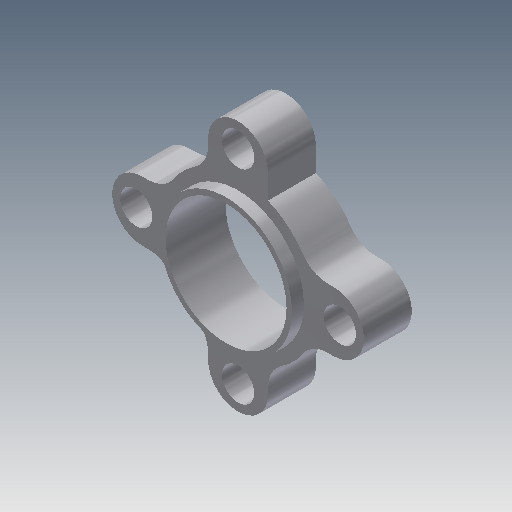
# Autodesk Inventor part: リンク_ふくらはぎ_サブフレーム_1_4
Saved by Autodesk Inventor 2017.3 (Build 213256000, 256)
## iProperties
Created: 2016-05-04
Part Number: リンク_ふくらはぎ_サブフレーム_1_4
Material: アルミニウム 2014-T4
Document SubType Name: Modeling
Designer: hiroaki
Density: 2.8 g/cm^3
Appearance: サテン
Mass: 1.21286 g
Surface Area: 8.00799 cm^2
Volume: 0.433165 cm^3
Author: hiroaki
Autodesk Inventor part; units mm, degrees
ref_plane "YZ Plane" through (0, 0, 0) normal (1, 0, 0) x (0, 1, 0)
ref_plane "XZ Plane" through (0, 0, 0) normal (0, 1, 0) x (-1, 0, 0)
ref_plane "XY Plane" through (0, 0, 0) normal (0, 0, 1) x (1, 0, 0)
sketch "スケッチ1" plane through (0, 0, 0) normal (0, 0, 1) x (1, 0, 0)
  circle A0 centre (0, 0) radius 10.5
  circle A1 centre (0, 0) radius 5.05
  circle A2 centre (0, 8.5) radius 1.35
  circle A3 centre (-6.0104, 6.0104) radius 1.04
  line L0 (0, 8.5) -> (0, 0) construction
  line L1 (0, 0) -> (-6.0104, 6.0104) construction
  circle A4 centre (0, 0) radius 8.5 construction
  circle A5 centre (-8.5, 0) radius 1.35
  circle A6 centre (-6.0104, -6.0104) radius 1.04
  circle A7 centre (0, -8.5) radius 1.35
  circle A8 centre (6.0104, -6.0104) radius 1.04
  circle A9 centre (8.5, 0) radius 1.35
  circle A10 centre (6.0104, 6.0104) radius 1.04
  dimension "d0" = 21
  dimension "d1" = 10.1
  dimension "d2" = 2.7
  dimension "d3" = 45
  dimension "d4" = 2.08
  dimension "d5" = 17
  dimension "d8" = 360
  constraints: 11 centre point, 4 coincident, 4 end point, 2 point on circle, 1 vertical, 1 vertical alignment, 17 other
  measures "d0" diameter of A0
  measures "d1" diameter of A1
  measures "d2" diameter of A2
  measures "d3" angle of L1 L0
  measures "d4" diameter of A3
  measures "d5" diameter of A4
extrude "押し出し1" add sketch "スケッチ1" along normal blind 4 contours A0 | A3 | A6 | A8 | A10
sketch "スケッチ2" plane through (0, 0, 4) normal (0, 0, 1) x (1, 0, 0)
  circle A0 centre (0, 0) radius 5.05 projected
  circle A1 centre (0, 0) radius 10.5 projected
  circle A2 centre (0, 0) radius 5.5
  dimension "d12" = 11
  constraints: 1 centre point, 1 coincident
  measures "d12" diameter of A2
extrude "押し出し2" add sketch "スケッチ2" along normal blind 1 contours A2
sketch "スケッチ4" plane through (0, 0, 4) normal (0, 0, 1) x (1, 0, 0)
  circle A0 centre (0, 0) radius 5.5 projected
  circle A1 centre (-8.5, 0) radius 1.35 projected
  circle A2 centre (0, 8.5) radius 1.35 projected
  circle A3 centre (0, 0) radius 10.5 projected
  line L0 (0, 8.5) -> (0, 0) construction
  line L1 (0, 0) -> (-8.5, 0) construction
  line L2 (0, 0) -> (-7.4246, 7.4246) construction
  circle A4 centre (0, 0) radius 10.5 construction
  line L3 (-12.2474, 2.5) -> (-6, 2.5)
  line L4 (-2.5, 6) -> (-2.5, 12.2474)
  arc A5 (-2.5, 12.2474) -> (-12.2474, 2.5) centre (0, 0) ccw
  arc A6 (-2.5, 6) -> (-6, 2.5) centre (0, 0) ccw
  circle A7 centre (0, 0) radius 5.5 projected
  line L5 (-2.5, -12.2474) -> (-2.5, -6)
  line L6 (-6, -2.5) -> (-12.2474, -2.5)
  arc A8 (-12.2474, -2.5) -> (-2.5, -12.2474) centre (0, 0) ccw
  arc A9 (-6, -2.5) -> (-2.5, -6) centre (0, 0) ccw
  line L7 (12.2474, -2.5) -> (6, -2.5)
  line L8 (2.5, -6) -> (2.5, -12.2474)
  arc A10 (2.5, -12.2474) -> (12.2474, -2.5) centre (0, 0) ccw
  arc A11 (2.5, -6) -> (6, -2.5) centre (0, 0) ccw
  line L9 (2.5, 12.2474) -> (2.5, 6)
  line L10 (6, 2.5) -> (12.2474, 2.5)
  arc A12 (12.2474, 2.5) -> (2.5, 12.2474) centre (0, 0) ccw
  arc A13 (6, 2.5) -> (2.5, 6) centre (0, 0) ccw
  dimension "d24" = 45
  dimension "d25" = 2.5
  dimension "d26" = 2.5
  dimension "d27" = 2
  dimension "d30" = 360
  dimension "d35" = 1
  constraints: 22 end point, 16 point on circle, 8 centre point, 2 coincident, 2 vertical, 1 horizontal, 1 perpendicular, 45 other
  measures "d24" angle of L0 L2
  measures "d25" distance between parallel lines of L1 L3
  measures "d26" distance between parallel lines of L0 L4
  measures "d35" radial gap between concentric circles of A0 A6
extrude "押し出し4" cut sketch "スケッチ4" against normal blind 10 contours L10 A13 L9 A3 | A3 L9 A12 L10 | L7 A10 L8 A3 | A3 L8 A11 L7 | L4 A6 L3 A3 | A3 L3 A5 L4 | L5 A8 L6 A3 | A3 L6 A9 L5
fillet "フィレット2" radius 2.5 15 edges at (2.5, -6, 2) (2.5, -10.198, 2) (-2.5, -10.198, 2) (-2.5, -6, 2) (6, -2.5, 2) (6, 2.5, 2) (10.198, -2.5, 2) (10.198, 2.5, 2) (2.5, 10.198, 2) (-2.5, 10.198, 2) (-2.5, 6, 2) (-6, 2.5, 2) (-10.198, -2.5, 2) (-10.198, 2.5, 2) (-6, -2.5, 2)
equation "\"d26\" = d25"
